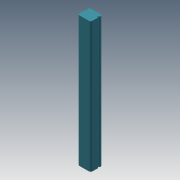
# Autodesk Inventor part: Rail-06
Saved by Autodesk Inventor 2014 (Build 180170000, 170)
## iProperties
Created: 2014-08-09
Part Number: Rail-06
Material: Generic
Document SubType Name: Modeling
Designer: Peele
Density: 1 g/cm^3
Appearance: Cadet Blue
Author: Peele
Autodesk Inventor part; units mm, degrees
ref_plane "YZ Plane" through (0, 0, 0) normal (1, 0, 0) x (0, 1, 0)
ref_plane "XZ Plane" through (0, 0, 0) normal (0, 1, 0) x (-1, 0, 0)
ref_plane "XY Plane" through (0, 0, 0) normal (0, 0, 1) x (1, 0, 0)
sketch "Sketch1" plane through (0, 0, 0) normal (0, 0, 1) x (1, 0, 0)
  line L0 (-7.5, -6.75) -> (7.5, -6.75)
  line L1 (7.5, -6.75) -> (7.5, 6.75)
  line L2 (7.5, 6.75) -> (-7.5, 6.75)
  line L3 (-7.5, 6.75) -> (-7.5, -6.75)
  line L4 (-7.5, -6.75) -> (7.5, 6.75) construction
  line L5 (7.5, -6.75) -> (-7.5, 6.75) construction
  point P0 (0, 0)
  dimension "d0" = 15
  dimension "d1" = 13.5
  constraints: 12 end point, 2 midpoint, 2 parallel, 1 horizontal, 1 perpendicular
  measures "d0" distance of L0.start L0.end
  measures "d1" distance of L2.end L0.start
extrude "Extrusion1" add sketch "Sketch1" along normal mid plane 150
sketch "Sketch2" plane through (0, 0, 75) normal (0, 0, 1) x (1, 0, 0)
  line L0 (7.5, 6.75) -> (-7.5, 6.75) projected
  line L1 (-7.5, 6.75) -> (-7.5, -6.75) projected
  line L2 (-7.5, 3.75) -> (-7, 3.25)
  line L3 (-7, 3.25) -> (-6.5, 3.25)
  line L4 (-6.5, 2.25) -> (-7, 2.25)
  line L5 (-7, 2.25) -> (-7.5, 1.75)
  arc A0 (-6.5, 2.25) -> (-6.5, 3.25) centre (-6.5, 2.75) ccw
  line L6 (-7.5, 1.75) -> (-7.5, 3.75)
  point P0 (0, 0)
  dimension "d4" = 4
  dimension "d5" = 1
  dimension "d6" = 0.5
  dimension "d7" = 0.5
  dimension "d8" = 2
  constraints: 10 end point, 2 equal length, 2 point on circle, 2 point on line, 2 tangent, 1 centre point, 1 collinear, 1 horizontal, 1 perpendicular
  measures "d4" distance from line of L0 A0.centre
  measures "d5" distance from line of L1 A0.centre
  measures "d6" distance of L2.end L3.end
  measures "d7" radius of A0
  measures "d8" distance of L5.end L2.start
extrude "Extrusion2" cut sketch "Sketch2" against normal up to next
mirror "Mirror1" about plane through (0, 0, 0) normal (1, 0, 0) of "Extrusion2"
fillet "Fillet1" radius 2 4 edges at (7.5, 6.75, 0) (-7.5, 6.75, 0) (7.5, -6.75, 0) (-7.5, -6.75, 0)
fillet "Fillet2" radius 1 8 edges at (-7, 2.25, 0) (-7.5, 1.75, 0) (-7, 3.25, 0) (-7.5, 3.75, 0) (7, 2.25, 0) (7.5, 1.75, 0) (7.5, 3.75, 0) (7, 3.25, 0)
body "Solid1"
